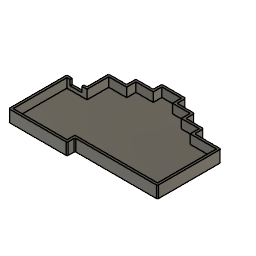
left_bottom (Autodesk Fusion 360 design; units mm, degrees)
part number: 2026-06-19-18-07-41-218
Autodesk Fusion 360 part; units mm, degrees
sketch "Sketch1" plane through (0, 0, 0) normal (0, 0, 1) x (1, 0, 0)
  line L0 (-77.1661, 21.8494) -> (-77.196, -36.9915)
  line L1 (-55.1143, 21.8382) -> (-77.1661, 21.8494)
  line L2 (-55.1022, 45.5931) -> (-55.1143, 21.8382)
  line L3 (-35.4199, 45.5831) -> (-55.1022, 45.5931)
  line L4 (-35.4199, 55.6506) -> (-35.4199, 45.5831)
  line L5 (-16.3374, 55.6581) -> (-35.4199, 55.6506)
  line L6 (-16.3374, 65.0231) -> (-16.3374, 55.6581)
  line L7 (5.0551, 65.0106) -> (-16.3374, 65.0231)
  line L8 (5.0551, 55.3606) -> (5.0551, 65.0106)
  line L9 (24.2287, 55.413) -> (5.0551, 55.3606)
  line L10 (24.2287, 45.8698) -> (24.2287, 55.413)
  line L11 (43.6774, 45.8599) -> (24.2287, 45.8698)
  line L12 (43.6724, 36.0748) -> (43.6774, 45.8599)
  line L13 (72.4097, 36.0602) -> (43.6724, 36.0748)
  line L14 (72.377, -28.4302) -> (72.4097, 36.0602)
  line L15 (-18.082, -28.4553) -> (72.377, -28.4302)
  line L16 (-18.0799, -36.9775) -> (-18.082, -28.4553)
  line L17 (-77.196, -36.9915) -> (-18.0799, -36.9775)
  line L18 (-18.8374, 67.5106) -> (7.5551, 67.5106)
  line L19 (7.5551, 67.5106) -> (7.5551, 57.913)
  line L20 (7.5551, 57.913) -> (26.7287, 57.913)
  line L21 (26.7287, 57.913) -> (26.7287, 48.3599)
  line L22 (26.7287, 48.3599) -> (46.1774, 48.3599)
  line L23 (46.1774, 48.3599) -> (46.1774, 38.5602)
  line L24 (74.9097, 38.5602) -> (46.1774, 38.5602)
  line L25 (74.9097, 38.5602) -> (74.8744, -30.9302)
  line L26 (-15.5799, -30.9553) -> (-15.5799, -39.4775)
  line L27 (-15.5799, -30.9553) -> (74.8744, -30.9302)
  line L28 (-15.5799, -39.4775) -> (-79.696, -39.4775)
  line L29 (-79.696, -39.4775) -> (-79.6636, 24.3382)
  line L30 (-79.6636, 24.3382) -> (-57.6022, 24.3382)
  line L31 (-57.6022, 24.3382) -> (-57.6022, 48.0931)
  line L32 (-57.6022, 48.0931) -> (-37.9199, 48.0931)
  line L33 (-37.9199, 58.1581) -> (-37.9199, 48.0931)
  line L34 (-37.9199, 58.1581) -> (-18.8374, 58.1581)
  line L35 (-18.8374, 58.1581) -> (-18.8374, 67.5106)
  dimension "d1" = 2.5
  dimension "d2" = 2.5
  dimension "d4" = 2.5
  dimension "d5" = 2.5
  dimension "d6" = 2.5
  dimension "d7" = 2.5
  dimension "d8" = 2.5
  dimension "d9" = 2.5
  dimension "d11" = 2.5
  dimension "d12" = 2.5
  dimension "d13" = 2.5
  dimension "d14" = 2.5
  dimension "d16" = 2.5
  dimension "d17" = 2.5
  dimension "d18" = 2.5
  dimension "d19" = 2.5
  dimension "d20" = 2.5
  dimension "d21" = 2.5
  dimension "d22" = 2.5
  constraint vertical L8
  constraint parallel L6 L8
  constraint vertical L4
  constraint perpendicular L2 L3
  constraint perpendicular L1 L2
  constraint perpendicular L0 L1
  constraint perpendicular L16 L17
  constraint perpendicular L1 L14
  constraint perpendicular L13 L14
  constraint perpendicular L12 L13
  constraint perpendicular L11 L14
  constraint vertical L10
  constraint perpendicular L6 L18
  constraint vertical L19
  constraint perpendicular L19 L20
  constraint perpendicular L20 L21
  constraint perpendicular L21 L22
  constraint perpendicular L22 L23
  constraint perpendicular L23 L24
  constraint coincident L23 L24.end
  constraint parallel L14 L25
  constraint vertical L26
  constraint horizontal L28
  constraint coincident L26 L28.start
  constraint parallel L0 L29
  constraint horizontal L30
  constraint coincident L29 L30.start
  constraint perpendicular L30 L31
  constraint coincident L30 L31.start
  constraint perpendicular L4 L32
  constraint vertical L33
  constraint coincident L31.end L32
  constraint coincident L32 L33.end
  constraint horizontal L34
  constraint perpendicular L34 L35
  constraint coincident L34 L35.start
  constraint coincident L33.start L34
  measures "d1" distance of L7.start L18
  measures "d2" horizontal distance of L7.start L18.end
  measures "d4" vertical distance of L9.start L19.end
  measures "d5" distance of L10 L21
  measures "d6" vertical distance of L11.start L22.end
  measures "d7" horizontal distance of L11.start L22.end
  measures "d8" vertical distance of L13.start L24.start
  measures "d9" horizontal distance of L13.start L24.start
  measures "d11" horizontal distance of L16.start L26.end
  measures "d12" vertical distance of L14.start L25.end
  measures "d13" vertical distance of L15.start L26.start
  measures "d14" vertical distance of L16.start L26.end
  measures "d16" horizontal distance of L0.end L28.end
  measures "d17" vertical distance of L1.start L30.end
  measures "d18" horizontal distance of L2.start L31.end
  measures "d19" vertical distance of L2.start L31.end
  measures "d20" horizontal distance of L4.start L33.start
  measures "d21" vertical distance of L5.start L34.end
  measures "d22" horizontal distance of L6.start L18.start
extrude "Extrude1" add sketch "Sketch1" along normal blind 13
extrude "Extrude2" add sketch "Sketch1" along normal blind 3 contours L0 L1 L2 L3 L4 L5 L6 L7 L8 L9 L10 L11 L12 L13 L14 L15 L16 L17
sketch "Sketch4" plane through (0, 0, 13) normal (0, 0, 1) x (-1, 0, 0)
  line L0 (18.0799, 36.9775) -> (77.196, 36.9915)
  line L1 (77.196, 36.9915) -> (77.1661, -21.8494)
  line L2 (77.1661, -21.8494) -> (55.1143, -21.8382)
  line L3 (55.1143, -21.8382) -> (55.1022, -45.5931)
  line L4 (55.1022, -45.5931) -> (35.4199, -45.5831)
  line L5 (35.4199, -45.5831) -> (35.4199, -55.6506)
  line L6 (35.4199, -55.6506) -> (16.3374, -55.6581)
  line L7 (16.3374, -55.6581) -> (16.3374, -65.0231)
  line L8 (16.3374, -65.0231) -> (-5.0551, -65.0106)
  line L9 (-5.0551, -65.0106) -> (-5.0551, -55.3606)
  line L10 (-5.0551, -55.3606) -> (-24.2287, -55.413)
  line L11 (-24.2287, -55.413) -> (-24.2287, -45.8698)
  line L12 (-24.2287, -45.8698) -> (-43.6774, -45.8599)
  line L13 (-43.6774, -45.8599) -> (-43.6724, -36.0748)
  line L14 (-43.6724, -36.0748) -> (-72.4097, -36.0602)
  line L15 (-72.4097, -36.0602) -> (-72.377, 28.4302)
  line L16 (-72.377, 28.4302) -> (18.082, 28.4553)
  line L17 (18.082, 28.4553) -> (18.0799, 36.9775)
  line L18 (37.9199, -58.1581) -> (37.9199, -48.0931)
  line L19 (37.9199, -48.0931) -> (57.6022, -48.0931)
  line L20 (57.6022, -48.0931) -> (57.6022, -24.3382)
  line L21 (57.6022, -24.3382) -> (79.6636, -24.3382)
  line L22 (79.6636, -24.3382) -> (79.696, 39.4775)
  line L23 (79.696, 39.4775) -> (15.5799, 39.4775)
  line L24 (15.5799, 39.4775) -> (15.5799, 30.9553)
  line L25 (15.5799, 30.9553) -> (-74.8744, 30.9302)
  line L26 (-74.8744, 30.9302) -> (-74.9097, -38.5602)
  line L27 (-74.9097, -38.5602) -> (-46.1774, -38.5602)
  line L28 (-46.1774, -38.5602) -> (-46.1774, -48.3599)
  line L29 (-46.1774, -48.3599) -> (-26.7287, -48.3599)
  line L30 (-26.7287, -48.3599) -> (-26.7287, -57.913)
  line L31 (-26.7287, -57.913) -> (-7.5551, -57.913)
  line L32 (-7.5551, -57.913) -> (-7.5551, -67.5106)
  line L33 (-7.5551, -67.5106) -> (18.8374, -67.5106)
  line L34 (18.8374, -67.5106) -> (18.8374, -58.1581)
  line L35 (18.8374, -58.1581) -> (37.9199, -58.1581)
  line L36 (73.8436, -24.8) -> (60.8436, -24.8)
  line L37 (60.8436, -24.8) -> (60.8436, -21.5)
  line L38 (60.8436, -21.5) -> (73.8436, -21.5)
  line L39 (73.8436, -21.5) -> (73.8436, -24.8)
  dimension "d27" = 13
  dimension "d28" = 5.82
  constraint horizontal L36
  constraint vertical L37
  constraint horizontal L38
  constraint vertical L39
  measures "d27" distance of L37 L39
  measures "d28" horizontal distance of L21.end L36.start
extrude "Extrude3" cut sketch "Sketch4" against normal blind 6 contours L2 L21 L37 L39
fillet "Fillet1" radius 1 18 edges at (-79.696, -39.4775, 6.5) (-15.5799, -39.4775, 6.5) (-15.5799, -30.9553, 6.5) (74.8744, -30.9302, 6.5) (74.9097, 38.5602, 6.5) (46.1774, 38.5602, 6.5) (26.7287, 48.3599, 6.5) (46.1774, 48.3599, 6.5) (26.7287, 57.913, 6.5) (7.5551, 67.5106, 6.5) (7.5551, 57.913, 6.5) (-57.6022, 48.0931, 6.5) (-57.6022, 24.3382, 6.5) (-79.6636, 24.3382, 6.5) (-37.9199, 48.0931, 6.5) (-37.9199, 58.1581, 6.5) (-18.8374, 58.1581, 6.5) (-18.8374, 67.5106, 6.5)
